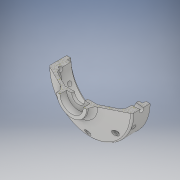
# Autodesk Inventor part: Drum
Saved by Autodesk Inventor 2018 (Build 220112000, 112)
## iProperties
Created: 2023-03-11
Part Number: Drum
Material: Generic
Document SubType Name: Modeling
Designer: Habib Mohamed
Density: 1 g/cm^3
Appearance: Default
Author: Habib Mohamed
Autodesk Inventor part; units mm, degrees
ref_plane "YZ Plane" through (0, 0, 0) normal (1, 0, 0) x (0, 1, 0)
ref_plane "XZ Plane" through (0, 0, 0) normal (0, 1, 0) x (-1, 0, 0)
ref_plane "XY Plane" through (0, 0, 0) normal (0, 0, 1) x (1, 0, 0)
sketch "Sketch1" plane through (0, 0, 0) normal (1, 0, 0) x (0, 1, 0)
  line L0 (0, 60.4181) -> (0, -60.4181) construction
  line L1 (14, 14.9983) -> (14, 6.9983)
  line L2 (14, 6.9983) -> (8, 6.9983)
  line L3 (8, 6.9983) -> (8, 3.4983)
  line L4 (8, 3.4983) -> (19.3103, 3.4983)
  line L5 (19.3103, 3.4983) -> (36.0783, -4.8876)
  line L6 (40.5, -12.0427) -> (40.5, -25.0017)
  line L7 (40.5, -25.0017) -> (45, -25.0017)
  line L8 (45, -25.0017) -> (45, -29.0017)
  line L9 (45, -29.0017) -> (50, -29.0017)
  line L10 (50, -29.0017) -> (50, -9.7905)
  line L11 (48.3419, -7.1074) -> (22.4217, 5.8555)
  line L12 (18, 13.0106) -> (18, 14.9983)
  line L13 (18, 14.9983) -> (14, 14.9983)
  arc A0 (18, 13.0106) -> (22.4217, 5.8555) centre (26, 13.0106) ccw
  arc A1 (50, -9.7905) -> (48.3419, -7.1074) centre (47, -9.7905) ccw
  arc A2 (40.5, -12.0427) -> (36.0783, -4.8876) centre (32.5, -12.0427) ccw
  point P0 (0, 0)
  point P1 (0, 0)
  dimension "d0" = 50
  dimension "d1" = 45
  dimension "d2" = 40.5
  dimension "d3" = 4
  dimension "d4" = 32.5
  dimension "d5" = 44
  dimension "d6" = 3.5
  dimension "d7" = 18
  dimension "d8" = 14
  dimension "d9" = 26.57
  dimension "d10" = 8
  dimension "d11" = 3.5
  dimension "d12" = 8
  dimension "d13" = 3
  constraints: 28 end point, 8 perpendicular, 6 point on circle, 6 tangent, 3 centre point, 3 parallel, 2 vertical, 1 coincident, 1 equal radius, 1 midpoint
  measures "d0" distance between parallel lines of L0 L10
  measures "d1" distance between parallel lines of L0 L8
  measures "d2" distance between parallel lines of L0 L6
  measures "d3" distance of L7.end L8.end
  measures "d4" distance between parallel lines of L4 L9
  measures "d5" distance between parallel lines of L9 L13
  measures "d6" distance between parallel lines of L11 L5
  measures "d7" distance between parallel lines of L12 L0
  measures "d8" distance between parallel lines of L0 L1
  measures "d9" angle of L9 L5
  measures "d10" distance between parallel lines of L0 L3
  measures "d11" distance between parallel lines of L2 L4
  measures "d12" radius of A0
  measures "d13" radius of A1
revolve "Revolution1" add sketch "Sketch1" angle 360 about axis through (0, 0, 60.4181) along (0, 0, -1)
sketch "Sketch2" plane through (0, 0, 0) normal (0, 1, 0) x (-1, 0, 0)
  circle A0 centre (9.21, -19.0017) radius 2.5
  circle A1 centre (-7, -12.5017) radius 2.5
  line L0 (0, -9.8686) -> (0, -47.9738) construction
  line L1 (-50, -29.0017) -> (50, -29.0017) projected
  point P0 (0, 0)
  dimension "d15" = 5
  dimension "d16" = 7
  dimension "d17" = 9.21
  dimension "d18" = 10
  dimension "d19" = 16.5
  constraints: 2 centre point, 2 end point, 1 equal radius, 1 point on line, 1 vertical
  measures "d15" diameter of A0
  measures "d16" distance from line of L0 A1.centre
  measures "d17" distance from line of L0 A0.centre
  measures "d18" distance from line of A0.centre L1
  measures "d19" distance from line of A1.centre L1
extrude "Extrusion1" cut sketch "Sketch2" along normal blind 59.5
sketch "Sketch3" plane through (0, 0, -25.0017) normal (0, 0, -1) x (-1, 0, 0)
  arc A0 (-9.4575, 39.3803) -> (-4.5425, 40.2444) centre (0, 0) ccw construction
  point P0 (0, 0)
  point P1 (0, -42.75)
  point P2 (0, -40.5)
  point P3 (0, -42.75)
  dimension "d22" = 2.25
  constraints: 2 vertical alignment, 1 coincident, 1 point on circle
  measures "d22" distance of point (0, -42.75) point (0, -40.5)
hole "Hole1" at (0, -42.75, -25.0017) direction (0, 0, 1) diameter 4 depth 24.5
sketch "Sketch4" plane through (0, 0, 0) normal (1, 0, 0) x (0, 1, 0)
  line L0 (-45, -25.0017) -> (45, -25.0017) construction
  line L1 (-42.75, -25.0017) -> (-42.75, 4.9936) construction
  line L2 (-42.75, -6.0017) -> (-39.25, -6.0017)
  line L3 (-39.25, -6.0017) -> (-39.25, -1.0017)
  line L4 (-39.25, -1.0017) -> (-42.75, -1.0017)
  line L5 (-42.75, -1.0017) -> (-42.75, -6.0017)
  line L6 (-40.75, -3.3106) -> (-40.75, -25.0017) construction
  line L7 (-40.75, -25.0017) -> (-44.75, -25.0017) construction
  line L8 (-44.75, -5.311) -> (-44.75, -25.0017) construction
  point P0 (0, 0)
  point P1 (-42.75, -25.0017)
  dimension "d30" = 3.5
  dimension "d31" = 19
  dimension "d32" = 5
  constraints: 12 end point, 7 point on line, 2 parallel, 1 horizontal, 1 midpoint, 1 perpendicular, 1 vertical
  measures "d30" distance of L3.end L4.end
  measures "d31" distance between parallel lines of L2 L0
  measures "d32" distance of L2.end L3.end
revolve "Revolution2" cut sketch "Sketch4" angle 360 about axis through (0, -42.75, -25.0017) along (0, 0, 1)
pattern_circular "Circular Pattern1" count 7 over 360 about axis through (0, 0, -19.3961) along (0, 0, -1) of "Extrusion1", "Hole1", "Revolution2"
equation "\"d11\" = d6"
body "Solid1"
